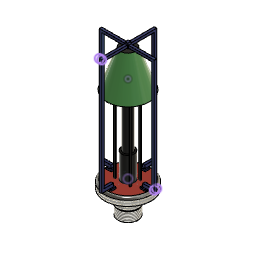
Buoyani-3D-v5 (Autodesk Fusion 360 design; units mm, degrees)
Autodesk Fusion 360 part; units mm, degrees
note: some values were not read from the file. Set by a fixed rule: which face or edge a step refers to.
sketch "Sketch1" plane through (0, 0, 0) normal (0, 0, 1) x (1, 0, 0)
  circle A0 centre (0, 0) radius 25
  dimension "d1" = 50
  constraint coincident A0.centre origin
  measures "d1" diameter of A0
extrude "Extrude1" add sketch "Sketch1" along normal blind 20 makes body 1
extrude "Extrude2" add 1 faces at (-6.7759, -1.242, 20) along direction (0, 0, 1) blind 10 on bodies 1 bodies 1
fillet "Fillet1" radius 4.5 1 faces at (-24.8758, 2.4892, 10) on bodies 1
extrude "Extrude3" add 1 faces at (5.4025, 6.3711, 30) along direction (0, 0, 1) blind 20 on bodies 1 bodies 1
sketch "Sketch2" plane through (0, 0, 50) normal (0, 0, 1) x (-1, 0, 0)
  circle A0 centre (0, 0) radius 20.5
  circle A1 centre (0, 0) radius 45
  dimension "d9" = 90
  constraint coincident A0.centre A1.centre
  measures "d9" diameter of A1
extrude "Extrude4" add sketch "Sketch2" along normal blind 20 separate body makes body 2
extrude "Extrude5" add 1 faces at (5.4025, 6.3711, 50) along direction (0, 0, 1) blind 100 on bodies 1 bodies 1 2
fillet "Fillet2" radius 7.5 1 edges at (41.9547, 16.2727, 70) on bodies 1
sketch "Sketch3" plane through (0, 0, 70) normal (0, 0, 1) x (-1, 0, 0)
  circle A0 centre (0, 0) radius 20.5
  circle A1 centre (0, 0) radius 37.5
  line L0 (-1, -29) -> (1, -29)
  line L1 (1, -29) -> (1, -31)
  line L2 (1, -31) -> (-1, -31)
  line L3 (-1, -31) -> (-1, -29)
  line L4 (-1, -29) -> (1, -31) construction
  line L5 (1, -29) -> (-1, -31) construction
  point P0 (0, -30)
  dimension "d15" = 2
  constraint horizontal L0
  constraint perpendicular L0 L1
  constraint parallel L0 L2
  constraint parallel L1 L3
  constraint coincident L4 P0
  constraint coincident L5 P0
  measures "d15" distance of L1.end L2.end
extrude "Extrude6" add sketch "Sketch3" along normal blind 100 contours L0 L1 L2 L3 bodies 1
move_face "MoveFace1" to x (0.939693, -0.34202, 0) y (0.34202, 0.939693, 0) z (0, 0, 1) at (-10.0558, 1.1527, 0) 1 faces at (0.3333, 29.6667, 170) on bodies 1
move_face "MoveFace2" by (1, -1, 0) 1 faces at (0.3333, 29.6667, 170) on bodies 1
sketch "Sketch4" plane through (0, 0, 70) normal (0, 0, 1) x (-1, 0, 0)
  line L0 (-1, -31) -> (-1, -29)
  line L1 (-1, -29) -> (1, -29)
  line L2 (1, -29) -> (1, -31)
  line L3 (1, -31) -> (-1, -31)
  circle A0 centre (0, 0) radius 20.5
  circle A1 centre (0, 0) radius 37.5
  line L4 (-1, 29) -> (1, 29)
  line L5 (1, 29) -> (1, 31)
  line L6 (1, 31) -> (-1, 31)
  line L7 (-1, 31) -> (-1, 29)
  line L8 (-1, 29) -> (1, 31) construction
  line L9 (1, 29) -> (-1, 31) construction
  point P0 (0, 30)
  dimension "d18" = 2
  constraint horizontal L4
  constraint perpendicular L4 L5
  constraint parallel L4 L6
  constraint parallel L5 L7
  constraint coincident L8 P0
  constraint coincident L9 P0
  measures "d18" distance of L4.end L5.end
extrude "Extrude7" add sketch "Sketch4" along normal blind 10 contours L4 L5 L6 L7 bodies 1
extrude "Extrude8" add 1 faces at (0.3333, -30.3333, 80) along direction (0, 0, 1) blind 90 on bodies 1 bodies 1
sketch "Sketch5" plane through (0, 0, 70) normal (0, 0, 1) x (-1, 0, 0)
  line L0 (-1, 31) -> (1, 31)
  line L1 (1, 31) -> (1, 29)
  line L2 (1, 29) -> (-1, 29)
  line L3 (-1, 29) -> (-1, 31)
  line L4 (-1, -31) -> (-1, -29)
  line L5 (-1, -29) -> (1, -29)
  line L6 (1, -29) -> (1, -31)
  line L7 (1, -31) -> (-1, -31)
  circle A0 centre (0, 0) radius 20.5
  circle A1 centre (0, 0) radius 37.5
  line L8 (29, -1) -> (31, -1)
  line L9 (31, -1) -> (31, 1)
  line L10 (31, 1) -> (29, 1)
  line L11 (29, 1) -> (29, -1)
  line L12 (29, -1) -> (31, 1) construction
  line L13 (31, -1) -> (29, 1) construction
  point P0 (30, 0)
  dimension "d23" = 2
  constraint horizontal L8
  constraint perpendicular L8 L9
  constraint parallel L8 L10
  constraint parallel L9 L11
  constraint coincident L12 P0
  constraint coincident L13 P0
  measures "d23" distance of L9.end L10.end
extrude "Extrude9" add sketch "Sketch5" along normal blind 100 contours L8 L9 L10 L11 bodies 1
sketch "Sketch6" plane through (0, 0, 70) normal (0, 0, 1) x (-1, 0, 0)
  line L0 (29, 1) -> (31, 1)
  line L1 (31, 1) -> (31, -1)
  line L2 (31, -1) -> (29, -1)
  line L3 (29, -1) -> (29, 1)
  line L4 (-1, 31) -> (1, 31)
  line L5 (1, 31) -> (1, 29)
  line L6 (1, 29) -> (-1, 29)
  line L7 (-1, 29) -> (-1, 31)
  line L8 (-1, -31) -> (-1, -29)
  line L9 (-1, -29) -> (1, -29)
  line L10 (1, -29) -> (1, -31)
  line L11 (1, -31) -> (-1, -31)
  circle A0 centre (0, 0) radius 20.5
  circle A1 centre (0, 0) radius 37.5
  line L12 (-31, -1) -> (-29, -1)
  line L13 (-29, -1) -> (-29, 1)
  line L14 (-29, 1) -> (-31, 1)
  line L15 (-31, 1) -> (-31, -1)
  line L16 (-31, -1) -> (-29, 1) construction
  line L17 (-29, -1) -> (-31, 1) construction
  point P0 (-30, 0)
  dimension "d26" = 2
  constraint horizontal L12
  constraint perpendicular L12 L13
  constraint parallel L12 L14
  constraint parallel L13 L15
  constraint coincident L16 P0
  constraint coincident L17 P0
  measures "d26" distance of L13.end L14.end
extrude "Extrude10" add sketch "Sketch6" along normal blind 100 contours L12 L13 L14 L15 bodies 1
sketch "Sketch7" plane through (0, 0, 150) normal (0, 0, 1) x (-1, 0, 0)
  circle A0 centre (0, 0) radius 20.5
  circle A1 centre (0, 0) radius 15
  dimension "d29" = 30
  constraint coincident A0.centre A1.centre
  measures "d29" diameter of A1
extrude "Extrude11" add sketch "Sketch7" along normal blind 200 contours A1 bodies 1
box "BoxPrimitive1" add length 3 width 6 height 1 placed x (0, -1, 0) y (1, 0, 0) z (0, 0, 1) at (20, 18, 70) bodies 1
box "BoxPrimitive2" add length 6 width 3 height 1 placed x (0, -1, 0) y (1, 0, 0) z (0, 0, 1) at (-27, 18, 70) bodies 1
box "BoxPrimitive3" add length 3 width 6 height 1 placed x (0, 1, 0) y (-1, 0, 0) z (0, 0, 1) at (-21, -20, 70) bodies 1
sketch "Sketch11" plane through (0, 0, 70) normal (0, 0, 1) x (-1, 0, 0)
  line L0 (21, 17) -> (21, 20)
  line L1 (21, 20) -> (27, 20)
  line L2 (27, 20) -> (27, 17)
  line L3 (27, 17) -> (21, 17)
  line L4 (27, -12) -> (27, -18)
  line L5 (27, -18) -> (24, -18)
  line L6 (24, -18) -> (24, -12)
  line L7 (24, -12) -> (27, -12)
  line L8 (-20, -15) -> (-20, -18)
  line L9 (-20, -18) -> (-26, -18)
  line L10 (-26, -18) -> (-26, -15)
  line L11 (-26, -15) -> (-20, -15)
  line L12 (-31, 1) -> (-29, 1)
  line L13 (-29, 1) -> (-29, -1)
  line L14 (-29, -1) -> (-31, -1)
  line L15 (-31, -1) -> (-31, 1)
  line L16 (29, 1) -> (31, 1)
  line L17 (31, 1) -> (31, -1)
  line L18 (31, -1) -> (29, -1)
  line L19 (29, -1) -> (29, 1)
  line L20 (-1, 31) -> (1, 31)
  line L21 (1, 31) -> (1, 29)
  line L22 (1, 29) -> (-1, 29)
  line L23 (-1, 29) -> (-1, 31)
  line L24 (-1, -31) -> (-1, -29)
  line L25 (-1, -29) -> (1, -29)
  line L26 (1, -29) -> (1, -31)
  line L27 (1, -31) -> (-1, -31)
  circle A0 centre (0, 0) radius 20.5
box "BoxPrimitive4" add length 6 width 3 height 1 placed x (0, 1, 0) y (-1, 0, 0) z (0, 0, 1) at (26, -20, 70) bodies 1
extrude "Extrude12" add 1 faces at (24, -18, 71) along direction (0, 0, 1) blind 250 on bodies 1 bodies 1
extrude "Extrude13" add 1 faces at (24, 17, 71) along direction (0, 0, 1) blind 250 on bodies 1 bodies 1
extrude "Extrude14" add 1 faces at (-25, -19, 71) along direction (0, 0, 1) blind 250 on bodies 1 bodies 1
extrude "Extrude15" add 1 faces at (-25, 16, 71) along direction (0, 0, 1) blind 250 on bodies 1 bodies 1
sketch "Sketch13" plane through (0, 0, 350) normal (0, 0, 1) x (-1, 0, 0)
  circle A0 centre (0, 0) radius 15
sketch "Sketch14" plane through (0, 0, 350) normal (0, 0, 1) x (-1, 0, 0)
extrude "Extrude16" cut sketch "Sketch13" against normal blind 30 bodies 1
sketch "Sketch15" plane through (0, 0, 320) normal (0, 0, 1) x (-1, 0, 0)
  circle A0 centre (0, 0) radius 15
  circle A1 centre (0, 0) radius 25
  dimension "d63" = 50
  constraint concentric A0 A1
  measures "d63" diameter of A1
extrude "Extrude17" add sketch "Sketch15" along normal blind 120 separate body makes body 3
draft "Draft1" angle 20 neutral plane through (0, 0, 440) pull (0, 0, 1) 1 faces at (24.8758, -2.4892, 360) on bodies 3
thread "Thread1" "ISO Metric profile 125.0 M125x8 6g" major diameter 124.545 minor diameter 115.3402 pitch 8 angle 60 resizes the face on face at (-44.7764, 4.4806, 54.1667) on bodies 1
thread "Thread2" "ISO Metric profile 70.0 M70x6 6g" major diameter 69.62 minor diameter 62.7358 pitch 6 angle 60 resizes the face on face at (24.9689, -1.2461, 18.5) on bodies 1
thread "Thread3" "ISO Metric profile 150.0 M150x8 6g" major diameter 149.545 minor diameter 140.3402 pitch 8 angle 60 resizes the face on face at (-62.1951, -3.104, 54.1667) on bodies 1
extrude "Extrude18" add 1 faces at (-1.862, -4.696, 0) along direction (0, 0, -1) blind 30 on bodies 1 bodies 1
thread "Thread4" "ISO Metric profile 65.0 M65x4 6g" major diameter 64.7025 minor diameter 60.1258 pitch 4 angle 60 resizes the face on face at (30.1594, 3.0179, -20) on bodies 1
extrude "Extrude19" add 1 faces at (-56.4033, -3.7148, 50) along direction (0, 0, -1) blind 5 on bodies 1 bodies 1
extrude "Extrude20" cut 1 faces at (0.3333, -30.3333, 170) along direction (0, 0, -1) blind 100 on bodies 1 bodies 1
extrude "Extrude21" cut 1 faces at (29.6667, 0.3333, 170) along direction (0, 0, -1) blind 100 on bodies 1 bodies 1
extrude "Extrude22" cut 1 faces at (-0.3333, 30.3333, 170) along direction (0, 0, -1) blind 100 on bodies 1 bodies 1
extrude "Extrude23" cut 1 faces at (-30.3333, 0.3333, 170) along direction (0, 0, -1) blind 100 on bodies 1 bodies 1
sketch "Sketch16" plane through (0, 0, 70) normal (0, 0, 1) x (-1, 0, 0)
  circle A0 centre (0, 0) radius 20.5
  line L0 (-20, -15) -> (-20, -18)
  line L1 (-20, -18) -> (-26, -18)
  line L2 (-26, -18) -> (-26, -15)
  line L3 (-26, -15) -> (-20, -15)
  line L4 (27, -12) -> (27, -18)
  line L5 (27, -18) -> (24, -18)
  line L6 (24, -18) -> (24, -12)
  line L7 (24, -12) -> (27, -12)
  line L8 (21, 17) -> (21, 20)
  line L9 (21, 20) -> (27, 20)
  line L10 (27, 20) -> (27, 17)
  line L11 (27, 17) -> (21, 17)
  line L12 (-26, 14) -> (-26, 20)
  line L13 (-26, 20) -> (-23, 20)
  line L14 (-23, 20) -> (-23, 14)
  line L15 (-23, 14) -> (-26, 14)
  circle A1 centre (0, 0) radius 67.2725
  line L16 (8, -47) -> (-8, -47)
  line L17 (-8, -47) -> (-8, -63)
  line L18 (-8, -63) -> (8, -63)
  line L19 (8, -63) -> (8, -47)
  line L20 (8, -47) -> (-8, -63) construction
  line L21 (-8, -47) -> (8, -63) construction
  line L22 (-47, 8) -> (-63, 8)
  line L23 (-63, 8) -> (-63, -8)
  line L24 (-63, -8) -> (-47, -8)
  line L25 (-47, -8) -> (-47, 8)
  line L26 (-47, 8) -> (-63, -8) construction
  line L27 (-63, 8) -> (-47, -8) construction
  line L28 (8, 63) -> (-8, 63)
  line L29 (-8, 63) -> (-8, 47)
  line L30 (-8, 47) -> (8, 47)
  line L31 (8, 47) -> (8, 63)
  line L32 (8, 63) -> (-8, 47) construction
  line L33 (-8, 63) -> (8, 47) construction
  line L34 (63, 8) -> (47, 8)
  line L35 (47, 8) -> (47, -8)
  line L36 (47, -8) -> (63, -8)
  line L37 (63, -8) -> (63, 8)
  line L38 (63, 8) -> (47, -8) construction
  line L39 (47, 8) -> (63, -8) construction
  point P0 (0, -55)
  point P1 (-55, 0)
  point P2 (0, 55)
  point P3 (55, 0)
  dimension "d80" = 16
  dimension "d81" = 16
  dimension "d82" = 16
  dimension "d83" = 16
  dimension "d84" = 16
  dimension "d85" = 16
  dimension "d86" = 16
  dimension "d87" = 16
  constraint horizontal L16
  constraint perpendicular L16 L17
  constraint parallel L16 L18
  constraint parallel L17 L19
  constraint coincident L20 P0
  constraint coincident L21 P0
  constraint horizontal L22
  constraint perpendicular L22 L23
  constraint parallel L22 L24
  constraint parallel L23 L25
  constraint coincident L26 P1
  constraint coincident L27 P1
  constraint horizontal L28
  constraint perpendicular L28 L29
  constraint parallel L28 L30
  constraint parallel L29 L31
  constraint coincident L32 P2
  constraint coincident L33 P2
  constraint horizontal L34
  constraint perpendicular L34 L35
  constraint parallel L34 L36
  constraint parallel L35 L37
  constraint coincident L38 P3
  constraint coincident L39 P3
  measures "d80" distance of L17.end L18.end
  measures "d81" distance of L16.end L17.end
  measures "d82" distance of L23.end L24.end
  measures "d83" distance of L22.end L23.end
  measures "d84" distance of L29.end L30.end
  measures "d85" distance of L28.end L29.end
  measures "d86" distance of L35.end L36.end
  measures "d87" distance of L34.end L35.end
extrude "Extrude24" add sketch "Sketch16" along normal blind 5 separate body contours L16 L17 L18 L19 | L22 L23 L24 L25 | L28 L29 L30 L31 | L34 L35 L36 L37 makes body 4 at (-52.3333, -2.6667, 70) makes body 5 at (2.6667, 52.3333, 70) makes body 6 at (2.6667, -57.6667, 70) makes body 7 at (57.6667, -2.6667, 70)
sketch "Sketch17" plane through (0, 0, 75) normal (0, 0, 1) x (-1, 0, 0)
  line L0 (63, -8) -> (63, 8)
  line L1 (63, 8) -> (47, 8)
  line L2 (47, 8) -> (47, -8)
  line L3 (47, -8) -> (63, -8)
  line L4 (59, 4) -> (51, 4)
  line L5 (51, 4) -> (51, -4)
  line L6 (51, -4) -> (59, -4)
  line L7 (59, -4) -> (59, 4)
  line L8 (59, 4) -> (51, -4) construction
  line L9 (51, 4) -> (59, -4) construction
  line L10 (4, -51) -> (-4, -51)
  line L11 (-4, -51) -> (-4, -59)
  line L12 (-4, -59) -> (4, -59)
  line L13 (4, -59) -> (4, -51)
  line L14 (4, -51) -> (-4, -59) construction
  line L15 (-4, -51) -> (4, -59) construction
  line L16 (-50.9781, 3.9059) -> (-58.9781, 3.9059)
  line L17 (-58.9781, 3.9059) -> (-58.9781, -4.0941)
  line L18 (-58.9781, -4.0941) -> (-50.9781, -4.0941)
  line L19 (-50.9781, -4.0941) -> (-50.9781, 3.9059)
  line L20 (-50.9781, 3.9059) -> (-58.9781, -4.0941) construction
  line L21 (-58.9781, 3.9059) -> (-50.9781, -4.0941) construction
  line L22 (4, 59) -> (-4, 59)
  line L23 (-4, 59) -> (-4, 51)
  line L24 (-4, 51) -> (4, 51)
  line L25 (4, 51) -> (4, 59)
  line L26 (4, 59) -> (-4, 51) construction
  line L27 (-4, 59) -> (4, 51) construction
  point P0 (55, 0)
  point P1 (0, -55)
  point P2 (-54.9781, -0.0941)
  point P3 (0, 55)
  dimension "d90" = 8
  dimension "d91" = 8
  dimension "d92" = 8
  dimension "d93" = 8
  dimension "d94" = 8
  dimension "d95" = 8
  dimension "d96" = 8
  dimension "d97" = 8
  constraint horizontal L4
  constraint perpendicular L4 L5
  constraint parallel L4 L6
  constraint parallel L5 L7
  constraint coincident L8 P0
  constraint coincident L9 P0
  constraint horizontal L10
  constraint perpendicular L10 L11
  constraint parallel L10 L12
  constraint parallel L11 L13
  constraint coincident L14 P1
  constraint coincident L15 P1
  constraint horizontal L16
  constraint perpendicular L16 L17
  constraint parallel L16 L18
  constraint parallel L17 L19
  constraint coincident L20 P2
  constraint coincident L21 P2
  constraint horizontal L22
  constraint perpendicular L22 L23
  constraint parallel L22 L24
  constraint parallel L23 L25
  constraint coincident L26 P3
  constraint coincident L27 P3
  measures "d90" distance of L5.end L6.end
  measures "d91" distance of L4.end L5.end
  measures "d92" distance of L11.end L12.end
  measures "d93" distance of L10.end L11.end
  measures "d94" distance of L17.end L18.end
  measures "d95" distance of L16.end L17.end
  measures "d96" distance of L23.end L24.end
  measures "d97" distance of L22.end L23.end
extrude "Extrude25" add sketch "Sketch17" along normal blind 10 contours L4 L5 L6 L7 | L10 L11 L12 L13 | L16 L17 L18 L19 | L22 L23 L24 L25 bodies 4 5 6 7
move_face "OffsetFaces1" offset 30 1 faces at (1.3333, 59, 78.3333) on bodies 5
move_face "OffsetFaces2" offset 30 1 faces at (-59, 1.3333, 78.3333) on bodies 4
move_face "OffsetFaces3" offset 30 1 faces at (-1.3333, -59, 78.3333) on bodies 6
move_face "OffsetFaces4" offset 30 1 faces at (58.9781, -1.2392, 78.3333) on bodies 7
sketch "Sketch18" plane through (0, 0, 70) normal (0, 0, 1) x (1, 0, 0)
delete_face "DeleteFace1" 1 faces at (-76.3333, -1.3333, 85) on bodies 4
sketch "Sketch19" plane through (0, 0, 85) normal (0, 0, 1) x (-1, 0, 0)
  line L0 (89, -4) -> (89, 4)
  line L1 (89, 4) -> (51, 4)
  line L2 (51, 4) -> (51, -4)
  line L3 (51, -4) -> (89, -4)
  line L4 (89, -4) -> (81, -4)
  line L5 (81, -4) -> (81, 4)
  line L6 (81, 4) -> (89, 4)
  line L7 (89, 4) -> (89, -4)
  line L8 (89, -4) -> (81, 4) construction
  line L9 (81, -4) -> (89, 4) construction
  point P0 (85, 0)
  constraint horizontal L4
  constraint perpendicular L4 L5
  constraint parallel L4 L6
  constraint parallel L5 L7
  constraint coincident L0.start L3.end
  constraint coincident L8 P0
  constraint coincident L9 P0
extrude "Extrude26" add sketch "Sketch19" along normal blind 100 contours L0 L1 L3 L4 L5 L6 L7 bodies 4
sketch "Sketch20" plane through (0, 0, 85) normal (0, 0, 1) x (-1, 0, 0)
  line L0 (4, -89) -> (4, -51)
  line L1 (4, -51) -> (-4, -51)
  line L2 (-4, -51) -> (-4, -89)
  line L3 (-4, -89) -> (4, -89)
  line L4 (4, -81) -> (-4, -81)
  line L5 (-4, -81) -> (-4, -89)
  line L6 (-4, -89) -> (4, -89)
  line L7 (4, -89) -> (4, -81)
  line L8 (4, -81) -> (-4, -89) construction
  line L9 (-4, -81) -> (4, -89) construction
  point P0 (0, -85)
  dimension "d108" = 8
  dimension "d109" = 8
  constraint horizontal L4
  constraint perpendicular L4 L5
  constraint parallel L4 L6
  constraint parallel L5 L7
  constraint coincident L8 P0
  constraint coincident L9 P0
  measures "d108" distance of L2.end L0.start
  measures "d109" distance of L4.end L2.end
extrude "Extrude27" add sketch "Sketch20" along normal blind 100 contours L0 L2 L3 L4 L5 L6 L7 bodies 5
sketch "Sketch21" plane through (0, 0, 85) normal (0, 0, 1) x (-1, 0, 0)
  line L0 (-50.9781, -4.0941) -> (-50.9781, 3.9059)
  line L1 (-50.9781, 3.9059) -> (-88.9781, 3.9059)
  line L2 (-88.9781, -4.0941) -> (-50.9781, -4.0941)
sketch "Sketch22" plane through (0, 0, 85) normal (0, 0, 1) x (-1, 0, 0)
  line L0 (-50.9781, -4.0941) -> (-50.9781, 3.9059)
  line L1 (-50.9781, 3.9059) -> (-88.9781, 3.9059)
  line L2 (-88.9781, 3.9059) -> (-88.9781, -4.0941)
  line L3 (-88.9781, -4.0941) -> (-50.9781, -4.0941)
  line L4 (-80.9781, 3.9059) -> (-88.9781, 3.9059)
  line L5 (-88.9781, 3.9059) -> (-88.9781, -4.0941)
  line L6 (-88.9781, -4.0941) -> (-80.9781, -4.0941)
  line L7 (-80.9781, -4.0941) -> (-80.9781, 3.9059)
  line L8 (-80.9781, 3.9059) -> (-88.9781, -4.0941) construction
  line L9 (-88.9781, 3.9059) -> (-80.9781, -4.0941) construction
  point P0 (-84.9781, -0.0941)
  dimension "d114" = 8
  dimension "d115" = 8
  constraint horizontal L4
  constraint perpendicular L4 L5
  constraint parallel L4 L6
  constraint parallel L5 L7
  constraint coincident L8 P0
  constraint coincident L9 P0
  constraint coincident L2.end L3.start
  measures "d114" distance of L2.end L6.end
  measures "d115" distance of L2.end L1.end
extrude "Extrude28" add sketch "Sketch22" along normal blind 100 contours L1 L2 L3 L4 L5 L6 L7 bodies 7
sketch "Sketch23" plane through (0, 0, 85) normal (0, 0, 1) x (-1, 0, 0)
  line L0 (4, 51) -> (4, 89)
  line L1 (4, 89) -> (-4, 89)
  line L2 (-4, 89) -> (-4, 51)
  line L3 (-4, 51) -> (4, 51)
  line L4 (4, 89) -> (-4, 89)
  line L5 (-4, 89) -> (-4, 81)
  line L6 (-4, 81) -> (4, 81)
  line L7 (4, 81) -> (4, 89)
  line L8 (4, 89) -> (-4, 81) construction
  line L9 (-4, 89) -> (4, 81) construction
  point P0 (0, 85)
  dimension "d118" = 8
  dimension "d119" = 8
  constraint horizontal L4
  constraint perpendicular L4 L5
  constraint parallel L4 L6
  constraint parallel L5 L7
  constraint coincident L8 P0
  constraint coincident L9 P0
  measures "d118" distance of L5.end L6.end
  measures "d119" distance of L1.end L5.end
extrude "Extrude29" add sketch "Sketch23" along normal blind 100 contours L0 L1 L2 L4 L5 L6 L7 bodies 6
extrude "Extrude30" add 1 faces at (-1.3333, -83.6667, 185) along direction (0, 0, 1) blind 100 on bodies 6 bodies 6
extrude "Extrude31" add 1 faces at (-1.3333, -83.6667, 285) along direction (0, 0, 1) blind 50 on bodies 6 bodies 6
extrude "Extrude32" add 1 faces at (-1.3333, -83.6667, 335) along direction (0, 0, 1) blind 110 on bodies 6 bodies 6
extrude "Extrude33" add 1 faces at (1.3333, 83.6667, 185) along direction (0, 0, 1) blind 260 on bodies 5 bodies 5
extrude "Extrude34" add 1 faces at (-83.6667, -1.3333, 185) along direction (0, 0, 1) blind 260 on bodies 4 bodies 4
extrude "Extrude35" add 1 faces at (83.6447, -1.2392, 185) along direction (0, 0, 1) blind 260 on bodies 7 bodies 7
extrude "Extrude36" add 1 faces at (-83.6667, -1.3333, 445) along direction (0, 0, 1) blind 10 on bodies 4 bodies 4
extrude "Extrude37" add 1 faces at (83.6447, -1.2392, 445) along direction (0, 0, 1) blind 10 on bodies 7 bodies 7
extrude "Extrude38" add 1 faces at (-1.3333, -83.6667, 445) along direction (0, 0, 1) blind 10 on bodies 6 bodies 6
extrude "Extrude39" add 1 faces at (1.3333, 83.6667, 445) along direction (0, 0, 1) blind 10 on bodies 5 bodies 5
extrude "Extrude40" add 1 faces at (-5.7141, -0.2203, 320) along direction (0, 0, 1) blind 120 on bodies 1 bodies 1 3
sketch "Sketch24" plane through (0, 0, 440) normal (0, 0, 1) x (-1, 0, 0)
  circle A0 centre (0, 0) radius 25
  line L0 (4, 4) -> (-4, 4)
  line L1 (-4, 4) -> (-4, -4)
  line L2 (-4, -4) -> (4, -4)
  line L3 (4, -4) -> (4, 4)
  line L4 (4, 4) -> (-4, -4) construction
  line L5 (-4, 4) -> (4, -4) construction
  dimension "d144" = 8
  dimension "d145" = 8
  constraint horizontal L0
  constraint perpendicular L0 L1
  constraint parallel L0 L2
  constraint parallel L1 L3
  constraint coincident L4 A0.centre
  constraint coincident L5 A0.centre
  constraint coincident A0.centre origin
  measures "d144" distance of L1.end L2.end
  measures "d145" distance of L0.end L1.end
extrude "Extrude41" add sketch "Sketch24" along normal blind 9 contours L0 L1 L2 L3 bodies 1
extrude "Extrude42" cut 1 faces at (1.3333, 83.6667, 455) along direction (0, 0, -1) blind 6 on bodies 5 bodies 5
extrude "Extrude43" cut 1 faces at (-83.6667, -1.3333, 455) along direction (0, 0, -1) blind 16 on bodies 4 bodies 4
extrude "Extrude44" cut 1 faces at (83.6447, -1.2392, 455) along direction (0, 0, -1) blind 6 on bodies 7 bodies 7
extrude "Extrude45" add 1 faces at (-83.6667, -1.3333, 439) along direction (0, 0, 1) blind 1 on bodies 4 bodies 4
extrude "Extrude46" add 1 faces at (-83.6667, -1.3333, 440) along direction (0, 0, 1) blind 1 on bodies 4 bodies 4
extrude "Extrude47" add 1 faces at (-83.6667, -1.3333, 441) along direction (0, 0, 1) blind 8 on bodies 4 bodies 4
extrude "Extrude48" cut 1 faces at (-1.3333, -83.6667, 455) along direction (0, 0, -1) blind 30 on bodies 6 bodies 6
extrude "Extrude49" add 1 faces at (-1.3333, -83.6667, 425) along direction (0, 0, 1) blind 10 on bodies 6 bodies 6
extrude "Extrude50" add 1 faces at (-1.3333, -83.6667, 435) along direction (0, 0, 1) blind 5 on bodies 6 bodies 6
extrude "Extrude51" add 1 faces at (-1.3333, -83.6667, 440) along direction (0, 0, 1) blind 5 on bodies 6 bodies 6
extrude "Extrude52" add 1 faces at (-1.3333, -83.6667, 445) along direction (0, 0, 1) blind 5 on bodies 6 bodies 6
sketch "Sketch25" plane through (-81, 0, 0) normal (1, 0, 0) x (0, 1, 0)
  line L0 (-4, 449) -> (-4, 85)
  line L1 (-4, 85) -> (4, 85)
  line L2 (4, 85) -> (4, 449)
  line L3 (4, 449) -> (-4, 449)
sketch "Sketch26" plane through (0, -89, 0) normal (0, -1, 0) x (1, 0, 0)
  line L0 (-4, 450) -> (-4, 75)
  line L1 (-4, 75) -> (4, 75)
  line L2 (4, 75) -> (4, 450)
extrude "Extrude53" add 1 faces at (1.3333, 83.6667, 449) along direction (0, 0, 1) blind 1 on bodies 5 bodies 5
sketch "Sketch27" plane through (0, -81, 0) normal (0, 1, 0) x (-1, 0, 0)
  line L0 (-4, 450) -> (-4, 85)
  line L1 (-4, 85) -> (4, 85)
  line L2 (4, 85) -> (4, 450)
  line L3 (4, 450) -> (-4, 450)
  line L4 (-4, 450) -> (4, 450)
  line L5 (4, 450) -> (4, 442)
  line L6 (4, 442) -> (-4, 442)
  line L7 (-4, 442) -> (-4, 450)
  line L8 (-4, 450) -> (4, 442) construction
  line L9 (4, 450) -> (-4, 442) construction
  point P0 (0, 446)
  dimension "d174" = 8
  dimension "d175" = 8
  constraint horizontal L4
  constraint perpendicular L4 L5
  constraint parallel L4 L6
  constraint parallel L5 L7
  constraint coincident L0.start L3.end
  constraint coincident L8 P0
  constraint coincident L9 P0
  measures "d174" distance of L5.end L6.end
  measures "d175" distance of L2.end L5.end
sketch "Sketch28" plane through (0, 81, 0) normal (0, -1, 0) x (1, 0, 0)
  line L0 (-4, 450) -> (-4, 85)
  line L1 (-4, 85) -> (4, 85)
  line L2 (4, 85) -> (4, 450)
  line L3 (4, 450) -> (-4, 450)
  line L4 (-4, 450) -> (4, 450)
  line L5 (4, 450) -> (4, 442)
  line L6 (4, 442) -> (-4, 442)
  line L7 (-4, 442) -> (-4, 450)
  line L8 (-4, 450) -> (4, 442) construction
  line L9 (4, 450) -> (-4, 442) construction
  point P0 (0, 446)
  dimension "d176" = 8
  dimension "d177" = 8
  constraint horizontal L4
  constraint perpendicular L4 L5
  constraint parallel L4 L6
  constraint parallel L5 L7
  constraint coincident L8 P0
  constraint coincident L9 P0
  measures "d176" distance of L5.end L6.end
  measures "d177" distance of L2.end L5.end
sketch "Sketch29" plane through (80.9781, 0, 0) normal (-1, 0, 0) x (0, -1, 0)
  line L0 (3.9059, 449) -> (-4.0941, 449)
  line L1 (-4.0941, 449) -> (-4.0941, 85)
  line L2 (-4.0941, 85) -> (3.9059, 85)
  line L3 (3.9059, 85) -> (3.9059, 449)
sketch "Sketch30" plane through (0, 0, 450) normal (0, 0, 1) x (-1, 0, 0)
  line L0 (4, 81) -> (4, 89)
  line L1 (4, 89) -> (-4, 89)
  line L2 (-4, 89) -> (-4, 81)
  line L3 (-4, 81) -> (4, 81)
delete_face "DeleteFace2" 1 faces at (4, -1.3333, 443) on bodies 1
move_face "OffsetFaces5" offset -0.1 1 faces at (-65, -4, 81.6667) on bodies 4
extrude "Extrude54" add sketch "Sketch27" along normal blind 75 contours L0 L2 L3 L4 L5 L6 L7 bodies 6
sketch "Sketch31" plane through (-81, 0, 267) normal (1, 0, 0) x (0, 1, 0)
  line L0 (-4, 182) -> (4, 182)
  line L1 (4, 182) -> (4, 174)
  line L2 (4, 174) -> (-4, 174)
  line L3 (-4, 174) -> (-4, 182)
  line L4 (-4, 182) -> (4, 174) construction
  line L5 (4, 182) -> (-4, 174) construction
  point P0 (0, 178)
  dimension "d183" = 8
  dimension "d184" = 8
  constraint horizontal L0
  constraint perpendicular L0 L1
  constraint parallel L0 L2
  constraint parallel L1 L3
  constraint coincident L4 P0
  constraint coincident L5 P0
  measures "d183" distance of L1.end L2.end
  measures "d184" distance of L0.end L1.end
move_face "OffsetFaces6" offset 0.1 1 faces at (-65, -3.9, 81.6667) on bodies 4
move_face "OffsetFaces7" offset 0.1 1 faces at (64.9854, -3.9059, 81.6667) on bodies 7
extrude "Extrude55" add sketch "Sketch31" along normal blind 75 bodies 4
move_face "OffsetFaces8" offset -0.1 1 faces at (-4, 65, 81.6667) on bodies 5
move_face "OffsetFaces9" offset 0.1 1 faces at (-3.9, 65, 81.6667) on bodies 5
extrude "Extrude56" add sketch "Sketch28" along normal blind 75 contours L0 L2 L3 L4 L5 L6 L7 bodies 5
sketch "Sketch32" plane through (80.9781, 0.0941, 267) normal (-1, 0, 0) x (0, -1, 0)
sketch "Sketch33" plane through (80.9781, 0.0941, 267) normal (-1, 0, 0) x (0, -1, 0)
  line L0 (4, 182) -> (-4, 182)
  line L1 (-4, 182) -> (-4, 174)
  line L2 (-4, 174) -> (4, 174)
  line L3 (4, 174) -> (4, 182)
  line L4 (4, 182) -> (-4, 174) construction
  line L5 (-4, 182) -> (4, 174) construction
  point P0 (0, 178)
  dimension "d193" = 8
  dimension "d194" = 8
  constraint horizontal L0
  constraint perpendicular L0 L1
  constraint parallel L0 L2
  constraint parallel L1 L3
  constraint coincident L4 P0
  constraint coincident L5 P0
  measures "d193" distance of L1.end L2.end
  measures "d194" distance of L0.end L1.end
extrude "Extrude57" cut 1 faces at (64.9854, -4.0059, 81.6667) along direction (0, 1, 0) blind 0.1 on bodies 7 bodies 7
extrude "Extrude58" add sketch "Sketch33" along normal blind 75 bodies 7
sketch "Sketch34" plane through (0, 0, 440) normal (0, 0, 1) x (-1, 0, 0)
  circle A0 centre (0, 0) radius 25
  line L0 (6, -6) -> (-6, -6)
  line L1 (-6, -6) -> (-6, 6)
  line L2 (-6, 6) -> (6, 6)
  line L3 (6, 6) -> (6, -6)
  line L4 (6, -6) -> (-6, 6) construction
  line L5 (-6, -6) -> (6, 6) construction
  dimension "d199" = 12
  dimension "d200" = 12
  constraint horizontal L0
  constraint perpendicular L0 L1
  constraint parallel L0 L2
  constraint parallel L1 L3
  constraint coincident L4 A0.centre
  constraint coincident L5 A0.centre
  constraint coincident A0.centre origin
  measures "d199" distance of L1.end L2.end
  measures "d200" distance of L0.end L1.end
extrude "Extrude59" add sketch "Sketch34" along normal blind 15 draft -5 separate body contours L0 L1 L2 L3 makes body 8
extrude "Extrude60" add 1 faces at (-6, -1.3333, 446.3333) along direction (1, 0, 0) blind 1 on bodies 4 bodies 4 8
extrude "Extrude61" add 1 faces at (5.9781, 1.4275, 446.3333) along direction (-1, 0, 0) blind 1 on bodies 7 bodies 7 4
extrude "Extrude62" add 1 faces at (-1.3333, 6, 444.6667) along direction (0, -1, 0) blind 1 on bodies 5 bodies 5 7
extrude "Extrude63" add 1 faces at (-1.3333, -6, 447.3333) along direction (0, 1, 0) blind 1 on bodies 6 bodies 6 5
